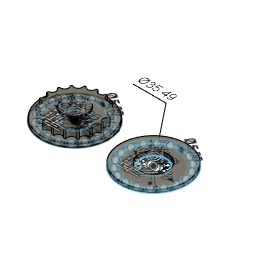
caveblind_ball.chain.pulley v1 (Autodesk Fusion 360 design; units mm, degrees)
Autodesk Fusion 360 part; units mm, degrees
sketch "Sketch1" plane through (0, 0, 0) normal (0, 1, 0) x (1, 0, 0)
  circle A0 centre (0, 0) radius 21
  circle A1 centre (0, 0) radius 17.4
  circle A2 centre (0, 0) radius 17.745
  line L0 (-1.8, -1.5) -> (1.8, -1.5)
  line L1 (3, -0.3) -> (3, 0.3)
  line L2 (1.8, 1.5) -> (-1.8, 1.5)
  line L3 (-3, 0.3) -> (-3, -0.3)
  line L4 (-3, -1.5) -> (3, 1.5) construction
  line L5 (3, -1.5) -> (-3, 1.5) construction
  arc A3 (-1.8, 1.5) -> (-3, 0.3) centre (-1.8, 0.3) ccw
  arc A4 (-3, -0.3) -> (-1.8, -1.5) centre (-1.8, -0.3) ccw
  arc A5 (1.8, -1.5) -> (3, -0.3) centre (1.8, -0.3) ccw
  arc A6 (3, 0.3) -> (1.8, 1.5) centre (1.8, 0.3) ccw
  circle A7 centre (0.0182, 17.745) radius 2.5
  circle A8 centre (0, 0) radius 8
  circle A9 centre (-6.052, 16.6811) radius 2.5
  circle A10 centre (-11.3923, 13.6052) radius 2.5
  circle A11 centre (-15.3585, 8.8883) radius 2.5
  circle A12 centre (-17.4722, 3.0993) radius 2.5
  circle A13 centre (-17.4786, -3.0635) radius 2.5
  circle A14 centre (-15.3767, -8.8567) radius 2.5
  circle A15 centre (-11.4202, -13.5817) radius 2.5
  circle A16 centre (-6.0863, -16.6686) radius 2.5
  circle A17 centre (-0.0182, -17.745) radius 2.5
  circle A18 centre (6.052, -16.6811) radius 2.5
  circle A19 centre (11.3923, -13.6052) radius 2.5
  circle A20 centre (15.3585, -8.8883) radius 2.5
  circle A21 centre (17.4722, -3.0993) radius 2.5
  circle A22 centre (17.4786, 3.0635) radius 2.5
  circle A23 centre (15.3767, 8.8567) radius 2.5
  circle A24 centre (11.4202, 13.5817) radius 2.5
  circle A25 centre (6.0863, 16.6686) radius 2.5
  circle A26 centre (67.4722, -3.0993) radius 2.5
  line L6 (47, 0.3) -> (47, -0.3)
  circle A27 centre (34.6233, -8.8567) radius 2.5
  line L7 (53, -1.5) -> (47, 1.5) construction
  arc A28 (48.2, 1.5) -> (47, 0.3) centre (48.2, 0.3) ccw
  circle A29 centre (49.9818, -17.745) radius 2.5
  line L8 (51.8, 1.5) -> (48.2, 1.5)
  line L9 (48.2, -1.5) -> (51.8, -1.5)
  arc A30 (51.8, -1.5) -> (53, -0.3) centre (51.8, -0.3) ccw
  circle A31 centre (34.6415, 8.8883) radius 2.5
  circle A32 centre (67.4786, 3.0635) radius 2.5
  circle A33 centre (38.6077, 13.6052) radius 2.5
  circle A34 centre (50, 0) radius 17.4
  arc A35 (53, 0.3) -> (51.8, 1.5) centre (51.8, 0.3) ccw
  circle A36 centre (56.0863, 16.6686) radius 2.5
  circle A37 centre (65.3585, -8.8883) radius 2.5
  arc A38 (47, -0.3) -> (48.2, -1.5) centre (48.2, -0.3) ccw
  line L10 (53, -0.3) -> (53, 0.3)
  circle A39 centre (43.9137, -16.6686) radius 2.5
  circle A40 centre (61.3923, -13.6052) radius 2.5
  circle A41 centre (56.052, -16.6811) radius 2.5
  circle A42 centre (50.0182, 17.745) radius 2.5
  circle A43 centre (65.3767, 8.8567) radius 2.5
  circle A44 centre (43.948, 16.6811) radius 2.5
  circle A45 centre (32.5278, 3.0993) radius 2.5
  circle A46 centre (50, 0) radius 8
  circle A47 centre (38.5798, -13.5817) radius 2.5
  line L11 (47, -1.5) -> (53, 1.5) construction
  circle A48 centre (32.5214, -3.0635) radius 2.5
  circle A49 centre (50, 0) radius 17.745
  circle A50 centre (50, 0) radius 21
  circle A51 centre (61.4202, 13.5817) radius 2.5
  point P0 (50, 0)
  point P1 (50, 0)
  dimension "d1" = 42
  dimension "d2" = 34.8
  dimension "d3" = 35.49
  dimension "d6" = 6
  dimension "d7" = 3
  dimension "d8" = 1.2
  dimension "d9" = 1.2
  dimension "d10" = 1.2
  dimension "d11" = 1.2
  dimension "d12" = 5
  dimension "d14" = 360
  dimension "d32" = 360
  dimension "d33" = 42
  dimension "d34" = 34.8
  dimension "d35" = 35.49
  dimension "d36" = 6
  dimension "d37" = 3
  dimension "d38" = 1.2
  dimension "d39" = 1.2
  dimension "d40" = 1.2
  dimension "d41" = 1.2
  dimension "d42" = 5
  constraint coincident A0.centre A1.centre
  constraint concentric A0 A2
  constraint horizontal L0
  constraint perpendicular L0 L1
  constraint parallel L0 L2
  constraint parallel L1 L3
  constraint coincident L4 A0.centre
  constraint coincident L5 A0.centre
  constraint coincident L5.end L2
  constraint coincident L5.end L3
  constraint tangent L2 A3
  constraint tangent L3 A3
  constraint coincident L4.start L3
  constraint coincident L4.start L0
  constraint tangent L3 A4
  constraint tangent L0 A4
  constraint coincident L5.start L0
  constraint coincident L5.start L1
  constraint tangent L0 A5
  constraint tangent L1 A5
  constraint coincident L4.end L1
  constraint coincident L4.end L2
  constraint tangent L1 A6
  constraint tangent L2 A6
  constraint coincident A2 A7.centre
  constraint coincident P1 P0
  constraint concentric A49 A50
  constraint horizontal L9
  constraint perpendicular L9 L10
  constraint parallel L8 L9
  constraint parallel L6 L10
  constraint coincident P1 L11
  constraint coincident P1 L7
  constraint coincident L7.end L8
  constraint coincident L7.end L6
  constraint tangent A28 L8
  constraint tangent L6 A28
  constraint coincident L11.start L6
  constraint coincident L11.start L9
  constraint tangent L6 A38
  constraint tangent L9 A38
  constraint coincident L7.start L9
  constraint coincident L7.start L10
  constraint tangent L9 A30
  constraint tangent A30 L10
  constraint coincident L11.end L10
  constraint coincident L11.end L8
  constraint tangent A35 L10
  constraint tangent L8 A35
  constraint coincident A42.centre A49
  measures "d1" diameter of A0
  measures "d2" diameter of A1
  measures "d3" diameter of A2
  measures "d6" distance of L4.end L5.end
  measures "d7" distance of L5.start L4.end
  measures "d8" radius of A3
  measures "d9" radius of A4
  measures "d10" radius of A5
  measures "d11" radius of A6
  measures "d12" diameter of A7
  measures "d33" diameter of A50
  measures "d34" diameter of A34
  measures "d35" diameter of A49
  measures "d36" distance of L11.end L7.end
  measures "d37" distance of L7.start L11.end
  measures "d38" radius of A28
  measures "d39" radius of A38
  measures "d40" radius of A30
  measures "d41" radius of A35
  measures "d42" diameter of A42
extrude "Extrude6" add sketch "Sketch1" along normal blind 2 contours A26 A49 | A26 A34 A49 | A26 A32 A34 A49 | A26 A34 A37 A49 | A26 A34 | A26 A27 A29 A31 A32 A33 A34 A36 A37 A39 A40 A41 A42 A43 A44 A45 A47 A48 A51 | A34 A37 A49 | A37 A49 | A32 A49 | A32 A34 A49 | A34 A37 | A34 A37 A40 A49 | A32 A34 | A32 A34 A43 A49 | A34 A40 A49 | A40 A49 | A43 A49 | A34 A43 A49 | A34 A40 | A34 A40 A41 A49 | A34 A43 | A34 A43 A49 A51 | A34 A41 A49 | A41 A49 | A34 A49 A51 | A49 A51 | A34 A41 | A29 A34 A41 A49 | A34 A51 | A34 A36 A49 A51 | A29 A34 A49 | A29 A49 | A36 A49 | A34 A36 A49 | A29 A34 | A29 A34 A39 A49 | A34 A36 | A34 A36 A42 A49 | A34 A39 A49 | A39 A49 | A42 A49 | A34 A42 A49 | A34 A39 | A34 A39 A47 A49 | A34 A42 | A34 A42 A44 A49 | A34 A47 A49 | A47 A49 | A44 A49 | A34 A44 A49 | A34 A47 | A27 A34 A47 A49 | A34 A44 | A33 A34 A44 A49 | A27 A34 A49 | A27 A49 | A33 A49 | A33 A34 A49 | A27 A34 | A27 A34 A48 A49 | A33 A34 | A31 A33 A34 A49 | A34 A48 A49 | A48 A49 | A31 A49 | A31 A34 A49 | A34 A48 | A34 A45 A48 A49 | A31 A34 | A31 A34 A45 A49 | A34 A45 A49 | A45 A49 | A34 A45 | A46 | A50 makes body 1
extrude "Extrude5" add sketch "Sketch1" along normal blind 1 from surface at 7 separate body contours A8 makes body 2
extrude "Extrude4" add sketch "Sketch1" along normal blind 5 from surface at 2 separate body contours A1 A7 A9 A10 A11 A12 A13 A14 A15 A16 A17 A18 A19 A20 A21 A22 A23 A24 A25 | A8 makes body 3
ref_plane "WorkPlane1" through (0, 2, 0) normal (0, 1, 0) x (-1, 0, 0)
ref_plane "WorkPlane2" through (0, 7, 0) normal (0, 1, 0) x (-1, 0, 0)
ref_plane "WorkPlane3" through (0, 9, 0) normal (0, 1, 0) x (-1, 0, 0)
extrude "Extrude1" add sketch "Sketch1" along normal blind 2 separate body contours A0 | A1 A7 A9 A10 A11 A12 A13 A14 A15 A16 A17 A18 A19 A20 A21 A22 A23 A24 A25 | A1 A2 A21 A22 | A1 A22 | A1 A2 A22 | A1 A2 A21 | A1 A21 | A1 A2 A22 A23 | A2 A22 | A1 A2 A20 A21 | A2 A21 | A1 A23 | A1 A2 A23 | A1 A2 A20 | A1 A20 | A1 A2 A23 A24 | A2 A23 | A1 A2 A19 A20 | A2 A20 | A1 A24 | A1 A2 A24 | A1 A2 A19 | A1 A19 | A1 A2 A24 A25 | A2 A24 | A1 A2 A18 A19 | A2 A19 | A1 A25 | A1 A2 A25 | A1 A2 A18 | A1 A18 | A1 A2 A7 A25 | A2 A25 | A1 A2 A17 A18 | A2 A18 | A1 A7 | A1 A2 A7 | A1 A2 A17 | A1 A17 | A1 A2 A7 A9 | A2 A7 | A1 A2 A16 A17 | A2 A17 | A1 A9 | A1 A2 A9 | A1 A2 A16 | A1 A16 | A1 A2 A9 A10 | A2 A9 | A1 A2 A15 A16 | A2 A16 | A1 A10 | A1 A2 A10 | A1 A2 A15 | A1 A15 | A1 A2 A10 A11 | A2 A10 | A1 A2 A14 A15 | A2 A15 | A1 A11 | A1 A2 A11 | A1 A2 A14 | A1 A14 | A1 A2 A11 A12 | A2 A11 | A1 A2 A13 A14 | A2 A14 | A1 A12 | A1 A2 A12 | A1 A2 A13 | A1 A13 | A1 A2 A12 A13 | A2 A12 | A2 A13 | A8 makes body 4
hole "Hole1" at (50, 2, 0) direction (0, -1, 0) diameter 18 depth 14 tip angle 180 bodies 1
fillet "Fillet1" radius 0.2 1 faces at (29.0261, 0.6667, -1.0468) on bodies 1
fillet "Fillet2" radius 0.2 1 faces at (50.8961, 1.3333, 8.9553) on bodies 1
fillet "Fillet3" radius 0.2 1 faces at (7.9602, 7.3333, 0.7965) on bodies 2
fillet "Fillet4" radius 0.02 1 faces at (-5.8225, 7, 9.1769) on bodies 3
fillet "Fillet5" radius 0.15 1 faces at (-20.9739, 0.6667, -1.0468) on bodies 4
named bodies: "base_plate", "chain holder", "top gap", "cover plate"
